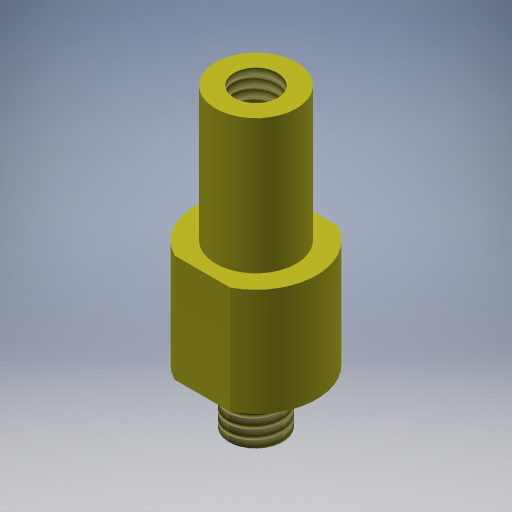
# Autodesk Inventor part: 24_0497_0022
Saved by Autodesk Inventor 2024.3 (Build 283343000, 343)
## iProperties
Created: 2024-07-08
Part Number: 24_0497_0022
Material: Allgemein
Document SubType Name: Modeling
Designer: Vogel
Density: 1 g/cm^3
Appearance: Kanariengelb
Author: Vogel
Autodesk Inventor part; units mm, degrees
ref_plane "YZ Plane" through (0, 0, 0) normal (1, 0, 0) x (0, 1, 0)
ref_plane "XZ Plane" through (0, 0, 0) normal (0, 1, 0) x (-1, 0, 0)
ref_plane "XY Plane" through (0, 0, 0) normal (0, 0, 1) x (1, 0, 0)
sketch "Skizze1" plane through (0, 0, 0) normal (0, 0, 1) x (1, 0, 0)
  line L0 (-6.3, 0) -> (6.3, 0) projected
  line L1 (0, -6.3) -> (0, 6.3) projected
  circle A0 centre (0, 0) radius 4.5
  dimension "d0" = 9
  constraints: 1 centre point, 1 coincident
  measures "d0" diameter of A0
extrude "Extrusion1" add sketch "Skizze1" along normal blind 8
sketch "Skizze2" plane through (0, 0, 0) normal (0, 0, -1) x (-1, 0, 0)
  circle A0 centre (0, 0) radius 4.5 projected
  circle A1 centre (0, 0) radius 2
  dimension "d3" = 4
  constraints: 1 centre point, 1 coincident
  measures "d3" diameter of A1
extrude "Extrusion2" add sketch "Skizze2" along normal blind 4 contours A1
thread "Gewinde1" size "M4x0.7" class "6g" standard "ANSI Metric M Profile" full length
sketch "Skizze3" plane through (0, 0, 8) normal (0, 0, 1) x (1, 0, 0)
  circle A0 centre (0, 0) radius 3
  dimension "d8" = 6
  constraints: 1 centre point, 1 coincident
  measures "d8" diameter of A0
extrude "Extrusion3" add sketch "Skizze3" along normal blind 10
sketch "Skizze4" plane through (0, 0, 8) normal (0, 0, 1) x (1, 0, 0)
  circle A0 centre (0, 0) radius 3 projected
  circle A1 centre (0, 0) radius 4.5 projected
  line L0 (-16.8, 0) -> (16.8, 0) projected
  line L1 (0, -6.3) -> (0, 6.3) projected
  line L2 (12, 4) -> (-12, 4)
  line L3 (-12, 4) -> (-12, -4)
  line L4 (-12, -4) -> (12, -4)
  line L5 (12, -4) -> (12, 4)
  line L6 (12, 4) -> (-12, -4) construction
  line L7 (-12, 4) -> (12, -4) construction
  point P0 (-2.0616, 4)
  point P1 (2.0616, 4)
  point P2 (-2.0616, -4)
  point P3 (2.0616, -4)
  dimension "d11" = 8
  constraints: 12 end point, 2 midpoint, 2 parallel, 1 horizontal, 1 perpendicular
  measures "d11" distance of L2.end L3.end
extrude "Extrusion4" cut sketch "Skizze4" against normal blind 10 contours L2 A1 L1 | L1 A1 L2 | L4 A1 L1 | L1 A1 L4
sketch "Skizze5" plane through (0, 0, 18) normal (0, 0, 1) x (1, 0, 0)
  circle A0 centre (0, 0) radius 2 projected
  constraints: 1 coincident
hole "Bohrung1" at (0, 0, 18) direction (0, 0, -1) diameter 3.242 depth 11.8 tip angle 118 thread size "M4x0.7" class "6H" standard "ISO Metric profile"
